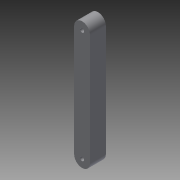
# Autodesk Inventor part: shortBar
Saved by Autodesk Inventor 2015 (Build 190159000, 159)
## iProperties
Created: 2015-04-09
Part Number: shortBar
Material: Generic
Document SubType Name: Modeling
Designer: WASHHSST
Density: 1 g/cm^3
Appearance: Default
Author: WASHHSST
Autodesk Inventor part; units mm, degrees
ref_plane "YZ Plane" through (0, 0, 0) normal (1, 0, 0) x (0, 1, 0)
ref_plane "XZ Plane" through (0, 0, 0) normal (0, 1, 0) x (-1, 0, 0)
ref_plane "XY Plane" through (0, 0, 0) normal (0, 0, 1) x (1, 0, 0)
sketch "Sketch1" plane through (0, 0, 0) normal (0, 1, 0) x (-1, 0, 0)
  line L0 (0, 0) -> (25.4, 0)
  line L1 (25.4, 0) -> (25.4, -25.4)
  line L2 (25.4, -25.4) -> (0, -25.4)
  line L3 (0, -25.4) -> (0, 0)
  dimension "d0" = 25.4
  dimension "d1" = 25.4
  constraints: 8 end point, 2 parallel, 1 horizontal, 1 perpendicular
  measures "d0" distance of L1.end L2.end
  measures "d1" distance of L0.end L1.end
extrude "Extrusion1" add sketch "Sketch1" along normal blind 203.2
hole "Hole1" at (-12.7, 190.5, 0) direction (0, 0, -1) diameter 6.35 end through all
ref_plane "Work Plane1" through (0, 101.6, 0) normal (0, 1, 0) x (1, 0, 0)
mirror "Mirror1" about plane through (0, 101.6, 0) normal (0, 1, 0) of "Hole1"
fillet "Fillet1" radius 12.7 4 edges at (0, 203.2, -12.7) (-25.4, 203.2, -12.7) (0, 0, -12.7) (-25.4, 0, -12.7)
body "Solid1"
